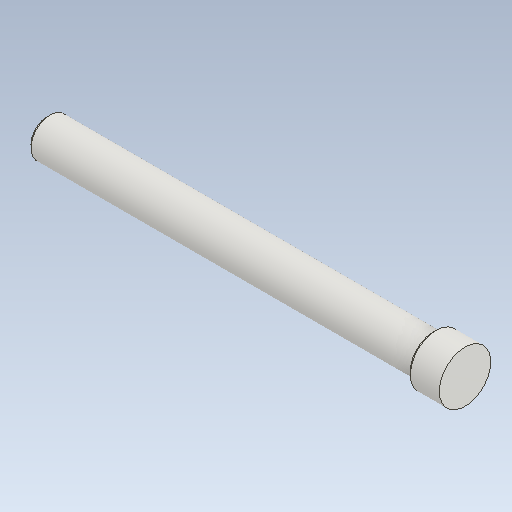
# Autodesk Inventor part: Shaft
Saved by Autodesk Inventor 2020 (Build 240168000, 168)
## iProperties
Created: 2020-03-25
Part Number: Shaft
Material: Steel
Document SubType Name: Modeling
Designer: Manish
Density: 1 g/cm^3
Appearance: Steel
CustomPartVersion: 1
Author: Manish
Length: 65.000 mm
d0: 0.000 mm
d1: 0.000 mm
d2: 0.00 deg
Autodesk Inventor part; units mm, degrees
ref_plane "Start Plane" through (0, 0, 0) normal (1, 0, 0) x (0, 1, 0)
ref_plane "XZ Plane" through (0, 0, 0) normal (0, 1, 0) x (-1, 0, 0)
ref_plane "XY Plane" through (0, 0, 0) normal (0, 0, 1) x (1, 0, 0)
sketch "Main Sketch" plane through (0, 0, 0) normal (0, 0, 1) x (1, 0, 0)
  line L0 (0, 0) -> (65, 0)
  line L1 (0, 0) -> (0, 3)
  line L2 (0, 3) -> (60, 3)
  line L3 (60, 3) -> (60, 4)
  line L4 (65, 4) -> (65, 0)
  line L5 (60, 4) -> (65, 4)
  dimension "d3" = 6
  dimension "d4" = 8
  constraints: 12 end point, 4 horizontal, 3 vertical
  measures "d3" diameter of L2 L0
  measures "d4" diameter of L5 L0
revolve "Revolution1" add sketch "Main Sketch" angle 360 about axis through (0, 0, 0) along (1, 0, 0)
chamfer "Chamfer1" distance 0.5 angle 45 1 edges at (0, -3, 0) measured on face at (40, 2.9903, -0.2414)
chamfer "Chamfer2" distance 0.5 angle 45 1 edges at (60, -4, 0) measured on face at (63.3333, 3.9482, -0.6416)
equation "\"Length\" = 65"
body "Solid1"
